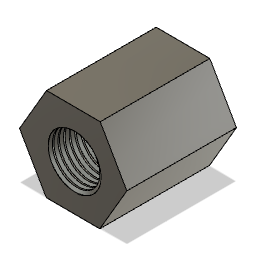
Converter part for pump (Autodesk Fusion 360 design; units mm, degrees)
Autodesk Fusion 360 part; units mm, degrees
sketch "M18 1.5mm" plane through (0, 0, 0) normal (0, 0, 1) x (1, 0, 0) in component "M18 1.5mm"
  circle A0 centre (0, 0) radius 9.5
  line L0 (-7.1611, 12.532) -> (-14.4336, 0.0643)
  line L1 (-14.4336, 0.0643) -> (-7.2725, -12.4677)
  line L2 (-7.2725, -12.4677) -> (7.1611, -12.532)
  line L3 (7.1611, -12.532) -> (14.4336, -0.0643)
  line L4 (14.4336, -0.0643) -> (7.2725, 12.4677)
  line L5 (7.2725, 12.4677) -> (-7.1611, 12.532)
  dimension "d2" = 19
  constraint coincident A0.centre origin
  measures "d2" diameter of A0
extrude "Extrude1" add sketch "M18 1.5mm" along normal blind 12 in component "M18 1.5mm"
sketch "M13 1.5mm" plane through (-6.4615, -0.389, 12) normal (0, 0, 1) x (1, 0, 0) in component "M18 1.5mm"
  circle A0 centre (6.4615, 0.389) radius 6.75
  line L0 (13.7339, 12.8567) -> (-0.6997, 12.921)
  line L1 (-0.6997, 12.921) -> (-7.9722, 0.4532)
  line L2 (-7.9722, 0.4532) -> (-0.811, -12.0788)
  line L3 (-0.811, -12.0788) -> (13.6226, -12.1431)
  line L4 (13.6226, -12.1431) -> (20.8951, 0.3247)
  line L5 (20.8951, 0.3247) -> (13.7339, 12.8567)
  line L6 (-0.7554, 12.889) -> (-7.9723, 0.389)
  line L7 (-7.9723, 0.389) -> (-0.7554, -12.111)
  line L8 (-0.7554, -12.111) -> (13.6783, -12.111)
  line L9 (13.6783, -12.111) -> (20.8952, 0.389)
  line L10 (20.8952, 0.389) -> (13.6783, 12.889)
  line L11 (13.6783, 12.889) -> (-0.7554, 12.889)
  circle A1 centre (6.4615, 0.389) radius 9.5
  point P0 (6.4615, 0.389)
  dimension "d5" = 13.5
  measures "d5" diameter of A0
extrude "Extrude2" add sketch "M13 1.5mm" along normal blind 17.5 contours A1 in component "M18 1.5mm"
thread "Thread4" "ISO Metric profile 15.0 M15x1.5 6H" major diameter 15.2033 minor diameter 13.5262 pitch 1.5 angle 60 modelled right hand crest width 0.4068 on face at (6.7165, -0.6721, 23.6667) crest through (6.7631, 0, 12.375) in component "M18 1.5mm"
extrude "Extrude3" add 1 faces at (0.2738, 11.4911, 12) along direction (0, 0, 1) blind 17.5 in component "M18 1.5mm"
thread "Thread5" "ISO Metric profile 20.0 M20x1.5 6H" major diameter 20.203 minor diameter 18.526 pitch 1.5 angle 60 modelled right hand crest width 0.4065 on face at (9.4882, -0.4735, 8) crest through (9.263, 0, 0.375) in component "M18 1.5mm"
component "M18 1.5mm" placed x (1, 0, 0) y (0, 1, 0) z (0, 0, 1) at (0, 0, 0)
